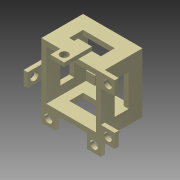
# Autodesk Inventor part: ygolki
Saved by Autodesk Inventor 2015 (Build 190159000, 159)
## iProperties
Created: 2016-05-14
Part Number: ygolki
Material: Nylon, molybdenum disulphide
Document SubType Name: Modeling
Designer: Andreas
Density: 1.13 g/cm^3
Appearance: Nylon 6
Author: Andreas
Autodesk Inventor part; units mm, degrees
ref_plane "YZ Plane" through (0, 0, 0) normal (1, 0, 0) x (0, 1, 0)
ref_plane "XZ Plane" through (0, 0, 0) normal (0, 1, 0) x (-1, 0, 0)
ref_plane "XY Plane" through (0, 0, 0) normal (0, 0, 1) x (1, 0, 0)
sketch "Sketch1" plane through (0, 0, 0) normal (0, 1, 0) x (-1, 0, 0)
  line L0 (0, 0) -> (0, -7)
  line L1 (0, -7) -> (2.5, -7)
  line L2 (2.5, -7) -> (2.5, -2.5)
  line L3 (2.5, -2.5) -> (7, -2.5)
  line L4 (7, -2.5) -> (7, 0)
  line L5 (7, 0) -> (0, 0)
  line L6 (0, -30) -> (0, -23)
  line L7 (0, -23) -> (2.5, -23)
  line L8 (2.5, -23) -> (2.5, -27.5)
  line L9 (2.5, -27.5) -> (7, -27.5)
  line L10 (7, -27.5) -> (7, -30)
  line L11 (7, -30) -> (0, -30)
  line L12 (23, 0) -> (30, 0)
  line L13 (30, 0) -> (30, -7)
  line L14 (30, -7) -> (27.5, -7)
  line L15 (27.5, -7) -> (27.5, -2.5)
  line L16 (27.5, -2.5) -> (23, -2.5)
  line L17 (23, -2.5) -> (23, 0)
  line L18 (30, -23) -> (30, -30)
  line L19 (30, -30) -> (23, -30)
  line L20 (23, -30) -> (23, -27.5)
  line L21 (23, -27.5) -> (27.5, -27.5)
  line L22 (27.5, -27.5) -> (27.5, -23)
  line L23 (27.5, -23) -> (30, -23)
  dimension "d0" = 7
  dimension "d1" = 2.5
  dimension "d2" = 4.5
  dimension "d3" = 4.5
  dimension "d8" = 7
  dimension "d9" = 4.5
  dimension "d10" = 7
  dimension "d11" = 7
  dimension "d12" = 2.5
  dimension "d13" = 30
  dimension "d14" = 30
  dimension "d15" = 30
  dimension "d16" = 2.5
  dimension "d17" = 2.5
  dimension "d18" = 4.5
  dimension "d19" = 7
  constraints: 48 end point, 16 perpendicular, 12 point on line, 2 vertical, 1 horizontal
  measures "d0" distance of L0.start L0.end
  measures "d1" distance of L0.end L1.end
  measures "d2" distance of L1.end L2.end
  measures "d3" distance of L2.end L3.end
  measures "d8" distance of L6.start L6.end
  measures "d9" distance of L7.end L8.end
  measures "d10" distance of L12.start L12.end
  measures "d11" distance of L12.end L13.end
  measures "d12" distance of L13.end L14.end
  measures "d13" distance of L0.start L12.end
  measures "d14" distance of L6.start L0.start
  measures "d15" distance of L6.start L18.end
  measures "d16" distance of L9.end L10.end
  measures "d17" distance of L6.end L7.end
  measures "d18" distance of L8.end L9.end
  measures "d19" distance of L10.end L6.start
extrude "Extrusion1" add sketch "Sketch1" along normal blind 20
sketch "Sketch2" plane through (0, 0, 0) normal (0, -1, 0) x (1, 0, 0)
  line L0 (0, 0) -> (-30, 0)
  line L1 (-30, 0) -> (-30, -30)
  line L2 (-30, -30) -> (0, -30)
  line L3 (0, -30) -> (0, 0)
  line L4 (-27.5, -2.5) -> (-2.5, -2.5)
  line L5 (-2.5, -2.5) -> (-2.5, -27.5)
  line L6 (-2.5, -27.5) -> (-27.5, -27.5)
  line L7 (-27.5, -27.5) -> (-23, -27.5) projected
  line L8 (-27.5, -27.5) -> (-27.5, -2.5)
  constraints: 16 end point, 5 perpendicular, 2 horizontal, 1 collinear
extrude "Extrusion2" add sketch "Sketch2" against normal blind 7
sketch "Sketch3" plane through (0, 20, 0) normal (0, 1, 0) x (1, 0, 0)
  line L0 (0, 0) -> (-7, 0)
  line L1 (0, 0) -> (-30, 0) projected
  line L2 (-7, 0) -> (-7, 7)
  line L3 (-7, 7) -> (0, 7)
  line L4 (0, 7) -> (0, 0)
  line L5 (0, 30) -> (-7, 30)
  line L6 (-7, 30) -> (-7, 23)
  line L7 (-7, 23) -> (0, 23)
  line L8 (-2.5, 23) -> (0, 23) projected
  line L9 (0, 23) -> (0, 30)
  line L10 (0, 23) -> (0, 30) projected
  line L11 (-30, 30) -> (-30, 23)
  line L12 (-30, 0) -> (-30, 30) projected
  line L13 (-30, 23) -> (-23, 23)
  line L14 (-23, 23) -> (-23, 30)
  line L15 (-23, 30) -> (-30, 30)
  line L16 (-30, 30) -> (0, 30) projected
  line L17 (-30, 0) -> (-23, 0)
  line L18 (-23, 0) -> (-23, 7)
  line L19 (-23, 7) -> (-30, 7)
  line L20 (-27.5, 7) -> (-30, 7) projected
  line L21 (-30, 7) -> (-30, 0)
  dimension "d24" = 7
  dimension "d25" = 7
  dimension "d26" = 7
  dimension "d27" = 7
  dimension "d28" = 7
  constraints: 32 end point, 5 collinear, 5 perpendicular, 3 point on line, 1 horizontal
  measures "d24" distance of L0.start L0.end
  measures "d25" distance of L0.end L2.end
  measures "d26" distance of L5.end L6.end
  measures "d27" distance of L11.start L11.end
  measures "d28" distance of L11.end L13.end
extrude "Extrusion3" add sketch "Sketch3" along normal blind 1
sketch "Sketch4" plane through (0, 0, 0) normal (1, 0, 0) x (0, 0, -1)
  line L0 (0, 0) -> (7, 0)
  line L1 (27.5, 0) -> (2.5, 0) projected
  line L2 (7, 0) -> (7, 2)
  line L3 (7, 2) -> (0, 2)
  line L4 (0, 2) -> (0, 0)
  line L5 (30, 0) -> (30, 2)
  line L6 (30, 0) -> (30, 21) projected
  line L7 (30, 2) -> (23, 2)
  line L8 (23, 2) -> (23, 0)
  line L9 (0, 0) -> (30, 0) projected
  line L10 (23, 0) -> (30, 0)
  dimension "d31" = 7
  dimension "d32" = 2
  dimension "d33" = 2
  dimension "d34" = 7
  constraints: 16 end point, 4 perpendicular, 3 point on line, 1 collinear, 1 vertical
  measures "d31" distance of L0.start L0.end
  measures "d32" distance of L0.end L2.end
  measures "d33" distance of L5.start L5.end
  measures "d34" distance of L5.end L7.end
sketch "Sketch5" plane through (0, 0, -30) normal (0, 0, -1) x (-1, 0, 0)
  line L0 (0, 0) -> (7, 0)
  line L1 (7, 0) -> (7, 2)
  line L2 (7, 2) -> (0, 2)
  line L3 (0, 2) -> (0, 0)
  line L4 (30, 0) -> (30, 2)
  line L5 (30, 0) -> (30, 21) projected
  line L6 (30, 2) -> (23, 2)
  line L7 (23, 2) -> (23, 0)
  line L8 (23, 0) -> (30, 0)
  line L9 (30, 0) -> (0, 0) projected
  dimension "d35" = 7
  dimension "d36" = 2
  dimension "d37" = 2
  dimension "d38" = 7
  constraints: 16 end point, 5 perpendicular, 1 collinear, 1 horizontal, 1 point on line
  measures "d35" distance of L0.start L0.end
  measures "d36" distance of L0.end L1.end
  measures "d37" distance of L4.start L4.end
  measures "d38" distance of L4.end L6.end
extrude "Extrusion4" add sketch "Sketch4" along normal blind 7
extrude "Extrusion5" add sketch "Sketch5" along normal blind 7
sketch "Sketch6" plane through (0, 2, 0) normal (0, 1, 0) x (1, 0, 0)
  circle A0 centre (3.5, 3.5) radius 2
  line L0 (7, 7) -> (7, 0) projected
  line L1 (0, 0) -> (7, 0) projected
  point P0 (7, 3.5)
  point P1 (3.5, 0)
  dimension "d43" = 4
  constraints: 2 midpoint, 1 centre point, 1 horizontal alignment, 1 vertical alignment
  measures "d43" diameter of A0
sketch "Sketch7" plane through (0, 2, -23) normal (0, 1, 0) x (1, 0, 0)
  circle A0 centre (3.5, 3.5) radius 2
  line L0 (7, 7) -> (7, 0) projected
  line L1 (0, 0) -> (7, 0) projected
  point P0 (0, -23)
  point P1 (7, 3.5)
  point P2 (3.5, 0)
  dimension "d44" = 4
  constraints: 2 midpoint, 1 centre point, 1 horizontal alignment, 1 vertical alignment
  measures "d44" diameter of A0
sketch "Sketch8" plane through (-7, 2, -30) normal (0, 1, 0) x (1, 0, 0)
  circle A0 centre (3.5, 3.5) radius 2
  circle A1 centre (-19.5, 3.5) radius 2
  line L0 (7, 0) -> (7, 7) projected
  line L1 (7, 0) -> (0, 0) projected
  line L2 (-23, 0) -> (-23, 7) projected
  line L3 (-23, 7) -> (-16, 7) projected
  point P0 (7, -30)
  point P1 (7, 3.5)
  point P2 (3.5, 0)
  point P3 (-23, 3.5)
  point P4 (-19.5, 7)
  dimension "d45" = 4
  dimension "d46" = 4
  constraints: 4 midpoint, 2 centre point, 2 horizontal alignment, 2 vertical alignment
  measures "d45" diameter of A0
  measures "d46" diameter of A1
extrude "Extrusion6" cut sketch "Sketch6" against normal blind 2
extrude "Extrusion7" cut sketch "Sketch7" against normal blind 2
extrude "Extrusion8" cut sketch "Sketch8" against normal blind 2
sketch "Sketch9" plane through (0, 21, 0) normal (0, 1, 0) x (1, 0, 0)
  line L0 (0, 30) -> (0, 0)
  line L1 (0, 0) -> (-30, 0)
  line L2 (7, 0) -> (-30, 0) projected
  line L3 (-30, 0) -> (-30, 30)
  line L4 (-30, 0) -> (-30, 37) projected
  line L5 (0, 30) -> (-30, 30)
  line L6 (-2.5, 27.5) -> (-27.5, 27.5)
  line L7 (-2.5, 27.5) -> (-27.5, 27.5) projected
  line L8 (-27.5, 27.5) -> (-27.5, 2.5)
  line L9 (-27.5, 2.5) -> (-2.5, 2.5)
  line L10 (-27.5, 2.5) -> (-2.5, 2.5) projected
  line L11 (-2.5, 2.5) -> (-2.5, 27.5)
  constraints: 16 end point, 3 collinear, 3 perpendicular, 1 point on line, 1 vertical
extrude "Extrusion9" add sketch "Sketch9" against normal blind 7
sketch "Sketch10" plane through (-30, 0, 0) normal (-1, 0, 0) x (0, 0, 1)
  line L0 (0, 0) -> (-11.5, 0)
  line L1 (-2.5, 0) -> (-27.5, 0) projected
  line L2 (-11.5, 0) -> (-11.5, -7)
  line L3 (-11.5, -7) -> (-18.5, -7)
  line L4 (-18.5, -7) -> (-18.5, 0)
  line L5 (-18.5, 0) -> (-18.5, 7)
  line L6 (-23, 7) -> (-7, 7) projected
  line L7 (-18.5, 7) -> (-11.5, 7)
  line L8 (-11.5, 0) -> (-11.5, 7)
  dimension "d55" = 11.5
  dimension "d56" = 7
  dimension "d57" = 7
  dimension "d58" = 7
  constraints: 14 end point, 5 point on line, 4 perpendicular
  measures "d55" distance of L0.start L0.end
  measures "d56" distance of L0.end L2.end
  measures "d57" distance of L2.end L3.end
  measures "d58" distance of L4.end L5.end
extrude "Extrusion10" add sketch "Sketch10" along normal blind 2
sketch "Sketch11" plane through (-30, 21, 0) normal (0, 0, 1) x (1, 0, 0)
  line L0 (0, -21) -> (11.5, -21)
  line L1 (7, -21) -> (23, -21) projected
  line L2 (11.5, -21) -> (18.5, -21)
  line L3 (18.5, -21) -> (18.5, -14)
  line L4 (7, -14) -> (23, -14) projected
  line L5 (18.5, -14) -> (11.5, -14)
  line L6 (11.5, -21) -> (11.5, -14)
  line L7 (11.5, -21) -> (11.5, -28)
  line L8 (11.5, -28) -> (18.5, -28)
  line L9 (18.5, -28) -> (18.5, -21)
  point P0 (30, -21)
  dimension "d61" = 11.5
  dimension "d62" = 7
  dimension "d63" = 7
  constraints: 16 end point, 5 point on line, 4 perpendicular
  measures "d61" distance of L0.start L0.end
  measures "d62" distance of L0.end L2.end
  measures "d63" distance of L0.end L7.end
extrude "Extrusion11" add sketch "Sketch11" along normal blind 2
sketch "Sketch12" plane through (-30, 21, 2) normal (0, 0, 1) x (1, 0, 0)
  circle A0 centre (15, -24.5) radius 2
  line L0 (18.5, -28) -> (18.5, -21) projected
  line L1 (11.5, -28) -> (18.5, -28) projected
  point P0 (30, -21)
  point P1 (18.5, -24.5)
  point P2 (15, -28)
  dimension "d66" = 4
  constraints: 2 midpoint, 1 centre point, 1 horizontal alignment, 1 vertical alignment
  measures "d66" diameter of A0
sketch "Sketch13" plane through (-32, 0, 0) normal (-1, 0, 0) x (0, 0, 1)
  circle A0 centre (-15, -3.5) radius 2
  line L0 (-11.5, -7) -> (-11.5, 0) projected
  line L1 (-18.5, -7) -> (-11.5, -7) projected
  point P0 (0, 0)
  point P1 (-11.5, -3.5)
  point P2 (-15, -7)
  dimension "d67" = 4
  constraints: 2 midpoint, 1 centre point, 1 horizontal alignment, 1 vertical alignment
  measures "d67" diameter of A0
extrude "Extrusion12" cut sketch "Sketch13" against normal blind 2
extrude "Extrusion13" cut sketch "Sketch12" against normal blind 2
body "Solid1"
